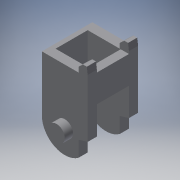
# Autodesk Inventor part: chain_elmt_2
Saved by Autodesk Inventor 2019.3 (Build 233278000, 278)
## iProperties
Created: 2020-08-28
Part Number: chain_elmt_2
Material: Generisch
Document SubType Name: Modeling
Designer: Nicolas Frick
Density: 1 g/cm^3
Appearance: Vorgabe
Author: Nicolas Frick
Autodesk Inventor part; units mm, degrees
ref_plane "YZ Plane" through (0, 0, 0) normal (1, 0, 0) x (0, 1, 0)
ref_plane "XZ Plane" through (0, 0, 0) normal (0, 1, 0) x (-1, 0, 0)
ref_plane "XY Plane" through (0, 0, 0) normal (0, 0, 1) x (1, 0, 0)
sketch "Skizze1" plane through (0, 0, 0) normal (0, 0, 1) x (1, 0, 0)
  arc A0 (5, -17) -> (-5, -17) centre (0, -17) ccw construction
  arc A1 (-5, -17) -> (3, -21) centre (0, -17) ccw
  circle A2 centre (0, -17) radius 1.75 construction
  line L0 (0, -22) -> (0, -4.9) construction
  line L1 (5, -17) -> (5, -4.9)
  line L2 (3, -4.9) -> (-5, -4.9)
  line L3 (-5, -4.9) -> (-5, -17)
  line L4 (0, -17) -> (3, -17) construction
  line L5 (3, -17.6027) -> (3, -21)
  line L6 (3, -17) -> (5, -17) construction
  line L7 (5, -17) -> (3, -17.6027)
  line L8 (3, -4.9) -> (3, -3.7947)
  line L9 (4, -2.9) -> (4.8065, -2.9)
  line L10 (5, -4.3512) -> (5, -4.9)
  line L11 (4, -2.9) -> (3, -3.7947)
  line L12 (4.8065, -2.9) -> (5, -4.3512)
  point P0 (0, 0)
  dimension "d0" = 3.5
  dimension "d1" = 17.1
  dimension "d2" = 3
  constraints: 26 end point, 3 perpendicular, 3 point on circle, 2 centre point, 2 coincident, 2 horizontal, 2 tangent, 2 vertical, 1 concentric, 1 parallel, 1 point on line
  measures "d0" diameter of A2
  measures "d1" distance of L0.start L0.end
  measures "d2" distance of L4.start L4.end
extrude "Extrusion1" add sketch "Skizze1" against normal blind 2
sketch "Skizze2" plane through (0, 0, 0) normal (0, 0, 1) x (1, 0, 0)
  arc A0 (-5, -17) -> (3, -21) centre (0, -17) ccw projected
  circle A1 centre (0, -17) radius 1.8
  point P0 (0, 0)
  dimension "d7" = 3.6
  constraints: 1 centre point, 1 coincident
  measures "d7" diameter of A1
extrude "Extrusion2" add sketch "Skizze2" along normal blind 1.8
sketch "Skizze4" plane through (0, 0, -2) normal (0, 0, -1) x (-1, 0, 0)
  line L0 (-5, -4.3512) -> (-5, -17) construction
  line L1 (-5, -17) -> (-3, -17.6027) construction
  line L2 (-3, -17.6027) -> (-3, -21) construction
  arc A0 (-3, -21) -> (5, -17) centre (0, -17) ccw construction
  line L3 (5, -17) -> (5, -4.9) construction
  line L4 (5, -4.9) -> (-3, -4.9) construction
  line L5 (-3, -4.9) -> (-3, -3.7947) construction
  line L6 (-3, -3.7947) -> (-4, -2.9) construction
  line L7 (-4, -2.9) -> (-4.8065, -2.9) construction
  line L8 (-4.8065, -2.9) -> (-5, -4.3512) construction
  line L9 (-5, -4.3512) -> (-5, -17) construction
  line L10 (-5, -4.9) -> (-3.2, -4.9)
  line L11 (-3.2, -4.9) -> (-3.2, -10.9)
  line L12 (-3.2, -10.9) -> (-5, -10.9)
  line L13 (-5, -10.9) -> (-5, -4.9)
  line L14 (-3, -4.9) -> (5, -4.9) construction
  line L15 (5, -4.9) -> (4, -4.9)
  line L16 (4, -4.9) -> (4, -13.7)
  line L17 (4, -13.7) -> (5, -13.7)
  line L18 (5, -13.7) -> (5, -4.9)
  point P0 (0, 0)
  dimension "d10" = 1.8
  dimension "d11" = 6
  dimension "d12" = 1
  dimension "d13" = 8.8
  constraints: 16 end point, 4 parallel, 2 horizontal, 2 perpendicular, 1 point on line
  measures "d10" distance of L11.end L12.end
  measures "d11" distance of L10.end L11.end
  measures "d12" distance of L17.end L16.end
  measures "d13" distance of L16.end L15.end
extrude "Extrusion3" add sketch "Skizze4" along normal blind 3.5
mirror "Spiegeln3" about plane through (4.1, -7.9, -5.5) normal (0, 0, -1) of "Extrusion2", "Extrusion1", "Extrusion3"
